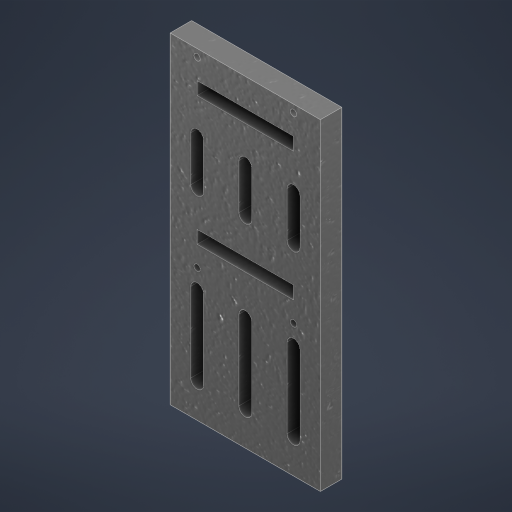
# Autodesk Inventor part: bay_mid
Saved by Autodesk Inventor 2023 (Build 270158000, 158)
## iProperties
Created: 2022-11-18
Part Number: bay_mid
Material: Generic
Document SubType Name: Modeling
Designer: washington
Density: 1 g/cm^3
Appearance: Fine Textured - Black
Author: washington
Autodesk Inventor part; units mm, degrees
ref_plane "YZ Plane" through (0, 0, 0) normal (1, 0, 0) x (0, 1, 0)
ref_plane "XZ Plane" through (0, 0, 0) normal (0, 1, 0) x (-1, 0, 0)
ref_plane "XY Plane" through (0, 0, 0) normal (0, 0, 1) x (1, 0, 0)
sketch "Sketch1" plane through (0, 0, 0) normal (0, 0, 1) x (1, 0, 0)
  line L0 (-35, 75) -> (35, 75)
  line L1 (35, 75) -> (35, -75)
  line L2 (35, -75) -> (-35, -75)
  line L3 (-35, -75) -> (-35, 75)
  line L4 (-35, 75) -> (35, -75) construction
  line L5 (35, 75) -> (-35, -75) construction
  circle A0 centre (-22.46, 71.46) radius 1.5
  circle A1 centre (22.46, 71.46) radius 1.5
  circle A2 centre (-22.46, -13.46) radius 1.5
  circle A3 centre (22.46, -13.46) radius 1.5
  line L6 (0, 18.5) -> (0, 39.5) construction
  line L7 (-3, 18.5) -> (-3, 39.5)
  line L8 (3, 39.5) -> (3, 18.5)
  arc A4 (-3, 18.5) -> (3, 18.5) centre (0, 18.5) ccw
  arc A5 (3, 39.5) -> (-3, 39.5) centre (0, 39.5) ccw
  line L9 (-11.23, 0) -> (-11.23, 75) construction
  line L10 (-19.46, 18.5) -> (-19.46, 39.5)
  line L11 (-25.46, 39.5) -> (-25.46, 18.5)
  arc A6 (-25.46, 18.5) -> (-19.46, 18.5) centre (-22.46, 18.5) ccw
  arc A7 (-19.46, 39.5) -> (-25.46, 39.5) centre (-22.46, 39.5) ccw
  line L12 (11.23, 0) -> (11.23, 75) construction
  line L13 (25.46, 18.5) -> (25.46, 39.5)
  line L14 (19.46, 39.5) -> (19.46, 18.5)
  arc A8 (19.46, 18.5) -> (25.46, 18.5) centre (22.46, 18.5) ccw
  arc A9 (25.46, 39.5) -> (19.46, 39.5) centre (22.46, 39.5) ccw
  line L15 (-22.46, 62) -> (22.46, 62)
  line L16 (22.46, 62) -> (22.46, 56)
  line L17 (22.46, 56) -> (-22.46, 56)
  line L18 (-22.46, 56) -> (-22.46, 62)
  line L19 (-22.46, 62) -> (22.46, 56) construction
  line L20 (22.46, 62) -> (-22.46, 56) construction
  line L21 (0, 29) -> (-22.46, 29) construction
  line L22 (-22.46, -4) -> (22.46, -4)
  line L23 (22.46, -4) -> (22.46, 2)
  line L24 (22.46, 2) -> (-22.46, 2)
  line L25 (-22.46, 2) -> (-22.46, -4)
  line L26 (0, -22.5) -> (0, -59.5) construction
  line L27 (-3, -22.5) -> (-3, -59.5)
  line L28 (3, -59.5) -> (3, -22.5)
  arc A10 (3, -22.5) -> (-3, -22.5) centre (0, -22.5) ccw
  arc A11 (-3, -59.5) -> (3, -59.5) centre (0, -59.5) ccw
  line L29 (-19.46, -22.5) -> (-19.46, -59.5)
  line L30 (-25.46, -59.5) -> (-25.46, -22.5)
  arc A12 (-19.46, -22.5) -> (-25.46, -22.5) centre (-22.46, -22.5) ccw
  arc A13 (-25.46, -59.5) -> (-19.46, -59.5) centre (-22.46, -59.5) ccw
  line L31 (25.46, -22.5) -> (25.46, -59.5)
  line L32 (19.46, -59.5) -> (19.46, -22.5)
  arc A14 (25.46, -22.5) -> (19.46, -22.5) centre (22.46, -22.5) ccw
  arc A15 (19.46, -59.5) -> (25.46, -59.5) centre (22.46, -59.5) ccw
  point P0 (0, 0)
  point P1 (0, 59)
  point P2 (0, -41)
  dimension "d0" = 3
  dimension "d1" = 22.46
  dimension "d2" = 3.54
  dimension "d5" = 44.92
  dimension "d8" = 84.92
  dimension "d11" = 150
  dimension "d12" = 70
  dimension "d13" = 42.46
  dimension "d14" = 31.96
  dimension "d15" = 22.46
  dimension "d16" = 3
  dimension "d17" = 11.23
  dimension "d18" = 22.46
  dimension "d19" = 44.92
  dimension "d20" = 6
  dimension "d21" = 59
  dimension "d22" = 22.5
  dimension "d23" = 37
  dimension "d24" = 6
  dimension "d25" = 75
  dimension "d26" = 75
  dimension "d27" = 57.46
  constraints: 70 end point, 28 symmetric about line, 24 point on circle, 16 centre point, 8 tangent, 6 midpoint, 6 parallel, 4 horizontal, 4 perpendicular, 3 vertical, 2 point on line, 2 vertical alignment, 14 other
  measures "d0" diameter of A0
  measures "d1" horizontal distance of A0.centre point (0, 0)
  measures "d2" distance from line of A0.centre L0
  measures "d5" distance of A0.centre A1.centre
  measures "d8" distance of A0.centre A2.centre
  measures "d11" distance of L0.end L1.end
  measures "d12" distance of L1.end L2.end
  measures "d13" vertical distance of L21.start A2.centre
  measures "d14" vertical distance of L6.start A2.centre
  measures "d15" horizontal distance of A3.centre L6.start
  measures "d16" radius of A5
  measures "d17" distance from line of L9 point (0, 0)
  measures "d18" distance between parallel lines of L12 L9
  measures "d19" distance of L15.start L15.end
  measures "d20" distance of L17.end L15.start
  measures "d21" distance of point (0, 59) point (0, 0)
  measures "d22" distance of point (0, 0) L26.start
  measures "d23" distance of L28.start L28.end
  measures "d24" distance between parallel lines of L28 L27
  measures "d25" distance from line of L12.start L0
  measures "d26" distance from line of L9.start L0
  measures "d27" distance from line of L21.end L1
extrude "Extrusion1" add sketch "Sketch1" against normal blind 10
body "Solid1"
